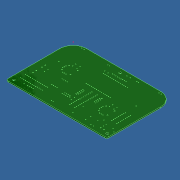
# Autodesk Inventor part: P1704_008_pcb
Saved by Autodesk Inventor 2019 (Build 230136000, 136)
## iProperties
Created: 2019-05-28
Part Number: P1704_008_pcb
Project: Nom Projet
Material: .
Description: Nom pièce
Document SubType Name: Modeling
Designer: Adel.KAHRIMANOVIC
Authority: brut Ø
Density: 0.001 g/cm^3
Appearance: Contour du circuit imprimé
Material number: ---
Author: Adel.KAHRIMANOVIC
Autodesk Inventor part; units mm, degrees
ref_plane "Plan YZ" through (0, 0, 0) normal (1, 0, 0) x (0, 1, 0)
ref_plane "Plan XZ" through (0, 0, 0) normal (0, 1, 0) x (-1, 0, 0)
ref_plane "Plan XY" through (0, 0, 0) normal (0, 0, 1) x (1, 0, 0)
sketch "Esquisse1" plane through (0, 0, 0) normal (0, 0, 1) x (1, 0, 0)
  point P0 (0, 0)
sketch "Esquisse6" plane through (0, 0, 0) normal (0, 0, 1) x (1, 0, 0)
  arc A0 (0, -97) -> (3, -100) centre (3, -97) ccw
  line L0 (3, -100) -> (147, -100)
  arc A1 (147, -100) -> (150, -97) centre (147, -97) ccw
  line L1 (150, -97) -> (150, -20)
  arc A2 (150, -20) -> (130, 0) centre (130, -20) ccw
  line L2 (130, 0) -> (20, 0)
  arc A3 (20, 0) -> (0, -20) centre (20, -20) ccw
  line L3 (0, -20) -> (0, -97)
  circle A4 centre (18.288, -55.88) radius 0.4
  circle A5 centre (18.288, -60.88) radius 0.4
  circle A6 centre (62.23, -15.24) radius 0.4
  circle A7 centre (67.23, -15.24) radius 0.4
  circle A8 centre (74.168, -72.136) radius 0.4
  circle A9 centre (74.168, -77.136) radius 0.4
  circle A10 centre (18.288, -91.44) radius 0.4
  circle A11 centre (23.288, -91.44) radius 0.4
  circle A12 centre (90.09, -5.08) radius 0.4
  circle A13 centre (85.09, -5.08) radius 0.4
  circle A14 centre (120.904, -94.488) radius 0.4
  circle A15 centre (120.904, -84.328) radius 0.4
  circle A16 centre (132.334, -83.185) radius 0.4
  circle A17 centre (142.494, -83.185) radius 0.4
  circle A18 centre (10.668, -52.07) radius 0.65
  circle A19 centre (10.668, -57.15) radius 0.65
  circle A20 centre (10.668, -65.532) radius 0.65
  circle A21 centre (10.668, -70.612) radius 0.65
  circle A22 centre (59.1922, -5.08) radius 0.4
  circle A23 centre (56.6522, -5.08) radius 0.4
  circle A24 centre (102.362, -5.08) radius 0.4
  circle A25 centre (99.822, -5.08) radius 0.4
  circle A26 centre (71.755, -13.335) radius 0.4
  circle A27 centre (74.295, -13.335) radius 0.4
  circle A28 centre (76.835, -13.335) radius 0.4
  circle A29 centre (79.375, -13.335) radius 0.4
  circle A30 centre (81.915, -13.335) radius 0.4
  circle A31 centre (84.455, -13.335) radius 0.4
  circle A32 centre (86.995, -13.335) radius 0.4
  circle A33 centre (89.535, -13.335) radius 0.4
  circle A34 centre (92.075, -13.335) radius 0.4
  circle A35 centre (137.414, -91.44) radius 0.65
  circle A36 centre (132.334, -91.44) radius 0.65
  circle A37 centre (60.325, -92.71) radius 0.4
  circle A38 centre (62.865, -92.71) radius 0.4
  circle A39 centre (96.266, -63.5) radius 0.4
  circle A40 centre (93.726, -62.23) radius 0.4
  circle A41 centre (96.266, -60.96) radius 0.4
  circle A42 centre (93.726, -59.69) radius 0.4
  circle A43 centre (96.266, -58.42) radius 0.4
  circle A44 centre (93.726, -57.15) radius 0.4
  circle A45 centre (96.266, -55.88) radius 0.4
  circle A46 centre (93.726, -54.61) radius 0.4
  circle A47 centre (69.85, -55.372) radius 0.4
  circle A48 centre (72.39, -56.642) radius 0.4
  circle A49 centre (69.85, -57.912) radius 0.4
  circle A50 centre (72.39, -59.182) radius 0.4
  circle A51 centre (69.85, -60.452) radius 0.4
  circle A52 centre (72.39, -61.722) radius 0.4
  circle A53 centre (69.85, -62.992) radius 0.4
  circle A54 centre (72.39, -64.262) radius 0.4
  circle A55 centre (68.326, -73.152) radius 0.4
  circle A56 centre (67.056, -75.692) radius 0.4
  circle A57 centre (65.786, -73.152) radius 0.4
  circle A58 centre (64.516, -75.692) radius 0.4
  circle A59 centre (63.246, -73.152) radius 0.4
  circle A60 centre (61.976, -75.692) radius 0.4
  circle A61 centre (60.706, -73.152) radius 0.4
  circle A62 centre (59.436, -75.692) radius 0.4
  circle A63 centre (26.75, -37.5) radius 0.45
  circle A64 centre (26.75, -40) radius 0.45
  circle A65 centre (26.75, -42.5) radius 0.45
  circle A66 centre (35, -48.25) radius 0.45
  circle A67 centre (32.5, -48.25) radius 0.45
  circle A68 centre (37.5, -48.25) radius 0.45
  circle A69 centre (31.75, -32.55) radius 0.4
  circle A70 centre (38.25, -32.55) radius 0.4
  circle A71 centre (38.25, -28.05) radius 0.4
  circle A72 centre (31.75, -28.05) radius 0.4
  circle A73 centre (111.75, -53.05) radius 0.4
  circle A74 centre (118.25, -53.05) radius 0.4
  circle A75 centre (118.25, -57.55) radius 0.4
  circle A76 centre (111.75, -57.55) radius 0.4
  circle A77 centre (117.5, -73.25) radius 0.45
  circle A78 centre (112.5, -73.25) radius 0.45
  circle A79 centre (115, -73.25) radius 0.45
  circle A80 centre (106.75, -67.5) radius 0.45
  circle A81 centre (106.75, -65) radius 0.45
  circle A82 centre (106.75, -62.5) radius 0.45
  circle A83 centre (110.236, -91.694) radius 0.4
  circle A84 centre (110.236, -84.074) radius 0.4
  circle A85 centre (132.334, -86.995) radius 0.4
  circle A86 centre (147.574, -86.995) radius 0.4
  circle A87 centre (124.968, -79.248) radius 0.4
  circle A88 centre (124.968, -94.488) radius 0.4
  circle A89 centre (91.948, -77.216) radius 0.4
  circle A90 centre (91.948, -92.456) radius 0.4
  circle A91 centre (15.75, -3) radius 0.5
  circle A92 centre (19.25, -3) radius 0.5
  circle A93 centre (15.75, -37) radius 0.5
  circle A94 centre (130.75, -3) radius 0.5
  circle A95 centre (134.25, -3) radius 0.5
  circle A96 centre (130.75, -37) radius 0.5
  circle A97 centre (100.205, -19.635) radius 0.4
  circle A98 centre (97.665, -19.635) radius 0.4
  circle A99 centre (95.125, -19.635) radius 0.4
  circle A100 centre (92.585, -19.635) radius 0.4
  circle A101 centre (90.045, -19.635) radius 0.4
  circle A102 centre (87.505, -19.635) radius 0.4
  circle A103 centre (84.965, -19.635) radius 0.4
  circle A104 centre (82.425, -19.635) radius 0.4
  circle A105 centre (79.885, -19.635) radius 0.4
  circle A106 centre (77.345, -19.635) radius 0.4
  circle A107 centre (74.805, -19.635) radius 0.4
  circle A108 centre (72.265, -19.635) radius 0.4
  circle A109 centre (69.725, -19.635) radius 0.4
  circle A110 centre (67.185, -19.635) radius 0.4
  circle A111 centre (64.645, -19.635) radius 0.4
  circle A112 centre (100.205, -45.135) radius 0.4
  circle A113 centre (72.265, -45.135) radius 0.4
  circle A114 centre (87.505, -45.135) radius 0.4
  circle A115 centre (77.345, -45.135) radius 0.4
  circle A116 centre (97.665, -45.135) radius 0.4
  circle A117 centre (92.585, -45.135) radius 0.4
  circle A118 centre (84.965, -45.135) radius 0.4
  circle A119 centre (74.805, -45.135) radius 0.4
  circle A120 centre (69.725, -45.135) radius 0.4
  circle A121 centre (90.045, -45.135) radius 0.4
  circle A122 centre (82.425, -45.135) radius 0.4
  circle A123 centre (67.185, -45.135) radius 0.4
  circle A124 centre (95.125, -45.135) radius 0.4
  circle A125 centre (64.645, -45.135) radius 0.4
  circle A126 centre (79.885, -45.135) radius 0.4
  circle A127 centre (7.62, -86.36) radius 0.4
  circle A128 centre (40.64, -78.74) radius 0.4
  circle A129 centre (10.16, -86.36) radius 0.4
  circle A130 centre (38.1, -78.74) radius 0.4
  circle A131 centre (12.7, -86.36) radius 0.4
  circle A132 centre (35.56, -78.74) radius 0.4
  circle A133 centre (15.24, -86.36) radius 0.4
  circle A134 centre (33.02, -78.74) radius 0.4
  circle A135 centre (17.78, -86.36) radius 0.4
  circle A136 centre (30.48, -78.74) radius 0.4
  circle A137 centre (20.32, -86.36) radius 0.4
  circle A138 centre (27.94, -78.74) radius 0.4
  circle A139 centre (22.86, -86.36) radius 0.4
  circle A140 centre (25.4, -78.74) radius 0.4
  circle A141 centre (25.4, -86.36) radius 0.4
  circle A142 centre (22.86, -78.74) radius 0.4
  circle A143 centre (27.94, -86.36) radius 0.4
  circle A144 centre (20.32, -78.74) radius 0.4
  circle A145 centre (30.48, -86.36) radius 0.4
  circle A146 centre (17.78, -78.74) radius 0.4
  circle A147 centre (33.02, -86.36) radius 0.4
  circle A148 centre (15.24, -78.74) radius 0.4
  circle A149 centre (35.56, -86.36) radius 0.4
  circle A150 centre (12.7, -78.74) radius 0.4
  circle A151 centre (38.1, -86.36) radius 0.4
  circle A152 centre (10.16, -78.74) radius 0.4
  circle A153 centre (40.64, -86.36) radius 0.4
  circle A154 centre (7.62, -78.74) radius 0.4
  circle A155 centre (79.756, -51.816) radius 0.4
  circle A156 centre (87.376, -84.836) radius 0.4
  circle A157 centre (79.756, -54.356) radius 0.4
  circle A158 centre (87.376, -82.296) radius 0.4
  circle A159 centre (79.756, -56.896) radius 0.4
  circle A160 centre (87.376, -79.756) radius 0.4
  circle A161 centre (79.756, -59.436) radius 0.4
  circle A162 centre (87.376, -77.216) radius 0.4
  circle A163 centre (79.756, -61.976) radius 0.4
  circle A164 centre (87.376, -74.676) radius 0.4
  circle A165 centre (79.756, -64.516) radius 0.4
  circle A166 centre (87.376, -72.136) radius 0.4
  circle A167 centre (79.756, -67.056) radius 0.4
  circle A168 centre (87.376, -69.596) radius 0.4
  circle A169 centre (79.756, -69.596) radius 0.4
  circle A170 centre (87.376, -67.056) radius 0.4
  circle A171 centre (79.756, -72.136) radius 0.4
  circle A172 centre (87.376, -64.516) radius 0.4
  circle A173 centre (79.756, -74.676) radius 0.4
  circle A174 centre (87.376, -61.976) radius 0.4
  circle A175 centre (79.756, -77.216) radius 0.4
  circle A176 centre (87.376, -59.436) radius 0.4
  circle A177 centre (79.756, -79.756) radius 0.4
  circle A178 centre (87.376, -56.896) radius 0.4
  circle A179 centre (79.756, -82.296) radius 0.4
  circle A180 centre (87.376, -54.356) radius 0.4
  circle A181 centre (79.756, -84.836) radius 0.4
  circle A182 centre (87.376, -51.816) radius 0.4
  circle A183 centre (131.572, -53.848) radius 0.4
  circle A184 centre (139.192, -74.168) radius 0.4
  circle A185 centre (131.572, -56.388) radius 0.4
  circle A186 centre (139.192, -71.628) radius 0.4
  circle A187 centre (131.572, -58.928) radius 0.4
  circle A188 centre (139.192, -69.088) radius 0.4
  circle A189 centre (131.572, -61.468) radius 0.4
  circle A190 centre (139.192, -66.548) radius 0.4
  circle A191 centre (131.572, -64.008) radius 0.4
  circle A192 centre (139.192, -64.008) radius 0.4
  circle A193 centre (131.572, -66.548) radius 0.4
  circle A194 centre (139.192, -61.468) radius 0.4
  circle A195 centre (131.572, -69.088) radius 0.4
  circle A196 centre (139.192, -58.928) radius 0.4
  circle A197 centre (131.572, -71.628) radius 0.4
  circle A198 centre (139.192, -56.388) radius 0.4
  circle A199 centre (131.572, -74.168) radius 0.4
  circle A200 centre (139.192, -53.848) radius 0.4
  circle A201 centre (48.26, -72.39) radius 0.45
  circle A202 centre (45.72, -72.39) radius 0.45
  circle A203 centre (43.18, -72.39) radius 0.45
  circle A204 centre (40.64, -72.39) radius 0.45
  circle A205 centre (40.64, -57.15) radius 0.45
  circle A206 centre (43.18, -57.15) radius 0.45
  circle A207 centre (45.72, -57.15) radius 0.45
  circle A208 centre (48.26, -57.15) radius 0.45
  circle A209 centre (26.71, -91.44) radius 0.4
  circle A210 centre (29.21, -91.44) radius 0.4
  circle A211 centre (31.71, -91.44) radius 0.4
  circle A212 centre (95.526, -53.21) radius 0.75
  circle A213 centre (70.59, -65.662) radius 0.75
  circle A214 centre (69.726, -74.952) radius 0.75
  circle A215 centre (28.75, -34.7) radius 0.65
  circle A216 centre (28.75, -45.3) radius 0.65
  circle A217 centre (41.25, -45.3) radius 0.65
  circle A218 centre (41.25, -34.7) radius 0.65
  circle A219 centre (121.25, -59.7) radius 0.65
  circle A220 centre (121.25, -70.3) radius 0.65
  circle A221 centre (108.75, -70.3) radius 0.65
  circle A222 centre (108.75, -59.7) radius 0.65
  circle A223 centre (76.2, -6.096) radius 1.6
  circle A224 centre (144.78, -93.98) radius 1.6
  circle A225 centre (6.096, -94.488) radius 1.6
  constraints: 226 centre point, 8 end point, 8 point on circle
extrude "manette_2019.kicad_pcb_Contour" add sketch "Esquisse6" along normal blind 1.6
